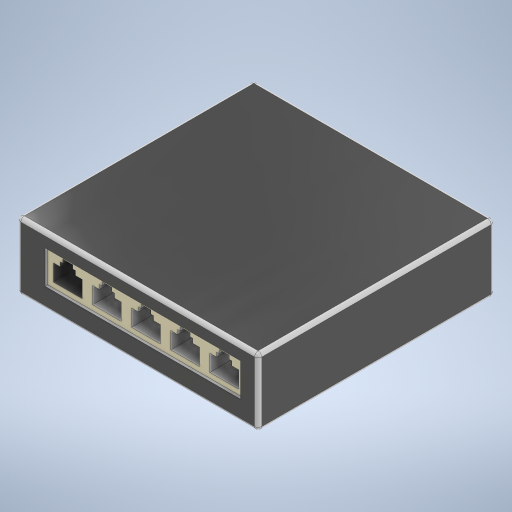
# Autodesk Inventor part: 5-port-switch
Saved by Autodesk Inventor 2023 (Build 270158030, 158C)
## iProperties
Created: 2024-03-26
Part Number: 5-port-switch
Material: Generic
Document SubType Name: Modeling
Designer: Imogen Heard
Density: 1 g/cm^3
Appearance: Default
Author: Imogen Heard
Autodesk Inventor part; units mm, degrees
ref_plane "YZ Plane" through (0, 0, 0) normal (1, 0, 0) x (0, 1, 0)
ref_plane "XZ Plane" through (0, 0, 0) normal (0, 1, 0) x (-1, 0, 0)
ref_plane "XY Plane" through (0, 0, 0) normal (0, 0, 1) x (1, 0, 0)
sketch "Sketch1" plane through (0, 0, 0) normal (0, 1, 0) x (-1, 0, 0)
  line L0 (50.2, -49.3) -> (-50.2, -49.3)
  line L1 (-50.2, -49.3) -> (-50.2, 49.3)
  line L2 (-50.2, 49.3) -> (50.2, 49.3)
  line L3 (50.2, 49.3) -> (50.2, -49.3)
  point P0 (0, 0)
  dimension "d0" = 100.4
  dimension "d1" = 98.6
  dimension "d2" = 49.3
  dimension "d3" = 50.2
  constraints: 8 end point, 2 parallel, 1 horizontal, 1 perpendicular
  measures "d0" distance between parallel lines of L1 L3
  measures "d1" distance between parallel lines of L2 L0
  measures "d2" distance from line of point (0, 0) L0
  measures "d3" distance from line of point (0, 0) L3
extrude "Extrusion1" add sketch "Sketch1" along normal blind 28.1
sketch "Sketch2" plane through (-50.2, 0, 49.3) normal (0, 0, 1) x (1, 0, 0)
  line L0 (11.65, 22.3) -> (93.1, 22.3)
  line L1 (93.1, 22.3) -> (93.1, 8.5)
  line L2 (93.1, 8.5) -> (11.65, 8.5)
  line L3 (11.65, 8.5) -> (11.65, 22.3)
  line L4 (100.4, 0) -> (100.4, 28.1) projected
  line L5 (0, 0) -> (0, 28.1) projected
  line L6 (0, 28.1) -> (100.4, 28.1) projected
  line L7 (0, 0) -> (100.4, 0) projected
  point P0 (50.2, 0)
  point P1 (100.4, 14.05)
  dimension "d6" = 7.3
  dimension "d7" = 11.65
  dimension "d8" = 5.8
  dimension "d9" = 8.5
  constraints: 8 end point, 2 parallel, 1 horizontal, 1 midpoint, 1 perpendicular
  measures "d6" distance from line of point (100.4, 14.05) L1
  measures "d7" distance between parallel lines of L5 L3
  measures "d8" distance between parallel lines of L6 L0
  measures "d9" distance between parallel lines of L7 L2
extrude "Extrusion2" cut sketch "Sketch2" against normal blind 1.08 contours L0 L1 L2 L3
sketch "Sketch3" plane through (-50.2, 0, 48.22) normal (0, 0, 1) x (1, 0, 0)
  line L0 (14, 17.6) -> (26, 17.6)
  line L1 (26, 17.6) -> (26, 10.65)
  line L2 (26, 10.65) -> (14, 10.65)
  line L3 (14, 10.65) -> (14, 17.6)
  line L4 (16.825, 19.4) -> (23.175, 19.4)
  line L5 (23.175, 19.4) -> (23.175, 17.6)
  line L6 (23.175, 17.6) -> (16.825, 17.6)
  line L7 (16.825, 17.6) -> (16.825, 19.4)
  line L8 (17.95, 20.92) -> (22.05, 20.92)
  line L9 (22.05, 20.92) -> (22.05, 19.4)
  line L10 (22.05, 19.4) -> (17.95, 19.4)
  line L11 (17.95, 19.4) -> (17.95, 20.92)
  line L12 (93.1, 8.5) -> (11.65, 8.5) projected
  line L13 (11.65, 8.5) -> (11.65, 22.3) projected
  point P0 (50.2, 0)
  point P1 (17.95, 19.4)
  dimension "d12" = 12
  dimension "d13" = 6.35
  dimension "d14" = 4.1
  dimension "d15" = 2.825
  dimension "d16" = 2.825
  dimension "d17" = 1.125
  dimension "d18" = 1.125
  dimension "d19" = 6.95
  dimension "d20" = 1.8
  dimension "d21" = 1.52
  dimension "d22" = 2.15
  dimension "d23" = 2.35
  constraints: 24 end point, 6 parallel, 3 horizontal, 3 perpendicular, 2 point on line
  measures "d12" distance between parallel lines of L1 L3
  measures "d13" distance between parallel lines of L5 L7
  measures "d14" distance between parallel lines of L9 L11
  measures "d15" distance between parallel lines of L3 L7
  measures "d16" distance between parallel lines of L1 L5
  measures "d17" distance between parallel lines of L7 L11
  measures "d18" distance between parallel lines of L5 L9
  measures "d19" distance between parallel lines of L2 L0
  measures "d20" distance between parallel lines of L0 L4
  measures "d21" distance between parallel lines of L4 L8
  measures "d22" distance between parallel lines of L12 L2
  measures "d23" distance between parallel lines of L13 L3
extrude "Extrusion3" cut sketch "Sketch3" against normal blind 11.78
pattern_linear "Rectangular Pattern1" count 5 spacing 16.3 along (1, 0, 0) of "Extrusion3"
fillet "Fillet1" radius 1.5 12 edges at (0, 28.1, -49.3) (-50.2, 28.1, 0) (0, 28.1, 49.3) (50.2, 28.1, 0) (50.2, 14.05, 49.3) (-50.2, 14.05, 49.3) (-50.2, 14.05, -49.3) (-50.2, 0, 0) (0, 0, -49.3) (50.2, 14.05, -49.3) (50.2, 0, 0) (0, 0, 49.3)
equation "\"d2\" = 0.5 * d1"
equation "\"d3\" = 0.5 * d0"
body "Solid1"
